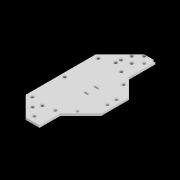
# Autodesk Inventor part: Placa Volante
Saved by Autodesk Inventor 2020 (Build 240168000, 168)
## iProperties
Created: 2022-11-26
Part Number: Placa Volante
Material: Genérico
Document SubType Name: Modeling
Designer: Alférez
Density: 1 g/cm^3
Appearance: Valor por defecto
Author: Alférez
Autodesk Inventor part; units mm, degrees
ref_plane "YZ Plane" through (0, 0, 0) normal (1, 0, 0) x (0, 1, 0)
ref_plane "XZ Plane" through (0, 0, 0) normal (0, 1, 0) x (-1, 0, 0)
ref_plane "XY Plane" through (0, 0, 0) normal (0, 0, 1) x (1, 0, 0)
sketch "Boceto1" plane through (0, 0, 0) normal (0, 1, 0) x (-1, 0, 0)
  line L0 (78, -28.2843) -> (49.7157, 0)
  line L1 (78, -129.6447) -> (42.6447, -165)
  line L2 (49.7157, 0) -> (29.7157, 0)
  line L3 (29.7157, 0) -> (29.7157, -30)
  line L4 (29.7157, -30) -> (0, -59.7157)
  line L5 (0, -59.7157) -> (0, -99.7157)
  line L6 (0, -99.7157) -> (25.4558, -125.1716)
  line L7 (0, -99.7157) -> (36, -99.7157) construction
  line L8 (78, -28.2843) -> (78, -129.6447)
  circle A0 centre (72, -78.6447) radius 2
  circle A1 centre (19.7157, -45) radius 2
  circle A2 centre (19.7157, -112) radius 2
  circle A3 centre (57.4939, -17.6777) radius 2
  circle A4 centre (52.5442, -140.9584) radius 2
  arc A5 (29.1447, -165) -> (25.4558, -163.5) centre (27.3714, -164.0751) ccw
  line L9 (29.1447, -165) -> (42.6447, -165)
  line L10 (25.4558, -125.1716) -> (25.4558, -163.5)
  point P0 (0, 0)
  dimension "d7" = 20
  dimension "d8" = 30
  dimension "d9" = 135
  dimension "d10" = 40
  dimension "d16" = 36
  dimension "d17" = 45
  dimension "d20" = 4
  dimension "d23" = 4
  dimension "d27" = 4
  dimension "d30" = 4
  dimension "d33" = 4
  dimension "d34" = 13.5
  constraints: 22 end point, 6 centre point, 2 horizontal, 2 point on circle, 1 equal length, 1 perpendicular, 1 vertical
  measures "d7" distance of L0.end L2.end
  measures "d8" distance of L2.end L3.end
  measures "d9" angle of L3 L4
  measures "d10" distance of L4.end L5.end
  measures "d16" distance of L5.end L6.end
  measures "d17" angle of L6 L7
  measures "d20" diameter of A0
  measures "d23" diameter of A1
  measures "d27" diameter of A2
  measures "d30" diameter of A3
  measures "d33" diameter of A4
  measures "d34" distance of L9.start L1.end
extrude "Extrusión1" add sketch "Boceto1" along normal blind 3
sketch "Boceto2" plane through (0, 0, 0) normal (0, -1, 0) x (1, 0, 0)
  circle A0 centre (-44.7157, -7.5) radius 2
  line L0 (-29.7157, 0) -> (-29.7157, -30) projected
  line L1 (-29.7157, -30) -> (-36.7157, -30)
  circle A1 centre (-36.7157, -30) radius 2
  line L2 (-36.7157, -30) -> (-70.2157, -30)
  circle A2 centre (-70.2157, -30) radius 2
  line L3 (-36.7157, -30) -> (-52.2157, -30)
  line L4 (-52.2157, -30) -> (-52.2157, -26.5)
  line L5 (0, -100.2087) -> (0, -87.7087)
  line L6 (0, -59.7157) -> (0, -99.7157) projected
  line L7 (0, -87.7087) -> (-6, -87.7087)
  line L8 (-6, -87.7087) -> (-6, -74.7087)
  circle A3 centre (-6, -87.7087) radius 2
  circle A4 centre (-6, -74.7087) radius 2
  line L9 (-25.4558, -125.1716) -> (-25.4558, -163.5) projected
  line L10 (-25.4558, -125.1716) -> (-25.4558, -153.4584)
  line L11 (-25.4558, -153.4584) -> (-31.4558, -153.4584)
  circle A5 centre (-31.4558, -153.4584) radius 2
  line L12 (-31.4558, -153.4584) -> (-49.4558, -153.4584)
  circle A6 centre (-49.4558, -153.4584) radius 2
  line L13 (-40.4558, -154.1716) -> (-40.4558, -145.1716)
  line L14 (-40.4558, -144.4584) -> (-40.4558, -162.4584)
  circle A7 centre (-40.4558, -162.4584) radius 2
  circle A8 centre (-40.4558, -144.4584) radius 2
  line L15 (-40.4558, -145.1716) -> (-40.4558, -133.6716)
  line L16 (-40.4558, -133.6716) -> (-37.4558, -133.6716)
  line L17 (-37.4558, -126.4584) -> (-70.9558, -126.4584)
  circle A9 centre (-70.9558, -126.4584) radius 2
  circle A10 centre (-37.4558, -126.4584) radius 2
  line L18 (-37.4558, -133.6716) -> (-52.9558, -133.6716)
  line L19 (-52.9558, -126.4584) -> (-52.9558, -129.9584)
  line L20 (-52.9558, -140.9584) -> (-52.9558, -129.9584)
  circle A11 centre (-52.9558, -133.6716) radius 2
  circle A12 centre (-52.5442, -140.9584) radius 2 projected
  line L21 (-52.5442, -140.9584) -> (-52.5442, -153.4584)
  line L22 (-52.5442, -153.4584) -> (-49.4558, -153.4584)
  circle A13 centre (-52.2157, -26.5) radius 2
  line L23 (-6, -81.2087) -> (0, -81.2087)
  line L24 (0, -81.2087) -> (-33, -81.2087)
  line L25 (-33, -81.2087) -> (-33, -73.2087)
  line L26 (-33, -73.2087) -> (-33, -89.2087)
  line L27 (-33, -89.2087) -> (-39, -89.2087)
  line L28 (-39, -89.2087) -> (-33, -89.2087)
  line L29 (-33, -89.2087) -> (-33, -73.2087)
  line L30 (-33, -73.2087) -> (-39, -73.2087)
  line L31 (-39, -73.2087) -> (-39, -89.2087)
  line L32 (-39, -89.2087) -> (-39, -87.7087)
  line L33 (-33, -73.2087) -> (-33, -74.7087)
  line L34 (-39, -87.7087) -> (-33, -87.7087)
  line L35 (-33, -87.7087) -> (-33, -74.7087)
  line L36 (-33, -74.7087) -> (-39, -74.7087)
  line L37 (-39, -74.7087) -> (-39, -87.7087)
  point P0 (0, 0)
  dimension "d43" = 4
  dimension "d44" = 7
  dimension "d45" = 4
  dimension "d46" = 33.5
  dimension "d47" = 4
  dimension "d48" = 15.5
  dimension "d49" = 3.5
  dimension "d50" = 12.5
  dimension "d51" = 6
  dimension "d52" = 13
  dimension "d53" = 4
  dimension "d54" = 4
  dimension "d58" = 4
  dimension "d60" = 4
  dimension "d63" = 4
  dimension "d64" = 4
  dimension "d66" = 3
  dimension "d67" = 33.5
  dimension "d68" = 4
  dimension "d69" = 4
  dimension "d70" = 15.5
  dimension "d71" = 3.5
  dimension "d72" = 11
  dimension "d73" = 4
  dimension "d74" = 12.5
  dimension "d75" = 4
  dimension "d76" = 33
  dimension "d77" = 8
  dimension "d78" = 16
  dimension "d79" = 6
  dimension "d80" = 1.5
  dimension "d81" = 1.5
  constraints: 70 end point, 13 centre point, 12 coincident, 11 perpendicular, 9 point on line, 5 horizontal, 5 parallel, 2 vertical, 1 collinear, 1 midpoint
  measures "d43" diameter of A0
  measures "d44" distance of L0.end L1.end
  measures "d45" diameter of A1
  measures "d46" distance of L2.start L2.end
  measures "d47" diameter of A2
  measures "d48" distance of L2.start L3.end
  measures "d49" distance of L3.end L4.end
  measures "d50" distance of L5.start L5.end
  measures "d51" distance of L5.end L7.end
  measures "d52" distance of L7.end L8.end
  measures "d53" diameter of A3
  measures "d54" diameter of A4
  measures "d58" diameter of A5
  measures "d60" diameter of A6
  measures "d63" diameter of A7
  measures "d64" diameter of A8
  measures "d66" distance of L16.end L15.end
  measures "d67" distance of L17.start L17.end
  measures "d68" diameter of A9
  measures "d69" diameter of A10
  measures "d70" distance of L18.start L18.end
  measures "d71" distance of L19.start L19.end
  measures "d72" distance of L20.start L20.end
  measures "d73" diameter of A11
  measures "d74" distance of L21.start L21.end
  measures "d75" diameter of A13
  measures "d76" distance of L23.end L24.end
  measures "d77" distance of L24.end L25.end
  measures "d78" distance of L25.end L26.end
  measures "d79" distance of L26.end L27.end
  measures "d80" distance of L27.end L32.end
  measures "d81" distance of L25.end L33.end
extrude "Extrusión2" cut sketch "Boceto2" against normal blind 10 contours A0 | A1 L2 L1 | L1 L2 A1 | A2 | A13 | A4 | A3 L8 L7 | L7 L8 A3 | L36 L31 L30 L25 | L26 L27 L31 L34 | A5 L12 L11 | L11 L12 A5 | A7 | A9 | A10 | A6 L22 L12 | L12 L22 A6 | A8 L15 L14 L13 | L13 L14 L15 A8 | A11 L20 L18 | L18 L20 A11 | L20 A11
